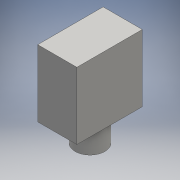
# Autodesk Inventor part: Toggle Switch
Saved by Autodesk Inventor 2016 (Build 200138000, 138)
## iProperties
Created: 2016-05-01
Part Number: Toggle Switch
Material: Generic
Document SubType Name: Modeling
Designer: Owner
Density: 1 g/cm^3
Appearance: Default
Author: Owner
Autodesk Inventor part; units mm, degrees
ref_plane "YZ Plane" through (0, 0, 0) normal (1, 0, 0) x (0, 1, 0)
ref_plane "XZ Plane" through (0, 0, 0) normal (0, 1, 0) x (-1, 0, 0)
ref_plane "XY Plane" through (0, 0, 0) normal (0, 0, 1) x (1, 0, 0)
sketch "Sketch1" plane through (0, 0, 0) normal (0, 0, 1) x (1, 0, 0)
  line L0 (0, 0) -> (7.9, 0)
  line L1 (7.9, 0) -> (7.9, 13.2)
  line L2 (7.9, 13.2) -> (0, 13.2)
  line L3 (0, 13.2) -> (0, 0)
  dimension "d0" = 7.9
  dimension "d1" = 13.2
  constraints: 8 end point, 2 parallel, 1 horizontal, 1 perpendicular
  measures "d0" distance of L2.end L1.end
  measures "d1" distance of L0.end L1.end
extrude "Extrusion1" add sketch "Sketch1" along normal blind 13.5
sketch "Sketch2" plane through (0, 0, 0) normal (0, 0, -1) x (-1, 0, 0)
  line L0 (-7.9, 13.2) -> (0, 13.2) projected
  line L1 (0, 13.2) -> (0, 0) projected
  circle A0 centre (-3.95, 6.6) radius 3
  point P0 (-3.95, 13.2)
  point P1 (0, 6.6)
  dimension "d4" = 6
  constraints: 2 midpoint, 1 centre point, 1 coincident
  measures "d4" diameter of A0
extrude "Extrusion2" add sketch "Sketch2" along normal blind 5
body "Solid1"
